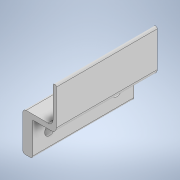
# Autodesk Inventor part: CableChain_Holder
Saved by Autodesk Inventor 2021 (Build 250183000, 183)
## iProperties
Created: 2021-12-04
Part Number: CableChain_Holder
Material: Generic
Document SubType Name: Modeling
Designer: Jorian Brusind
Density: 1 g/cm^3
Appearance: Default
Author: Jorian Brusind
Autodesk Inventor part; units mm, degrees
ref_plane "YZ Plane" through (0, 0, 0) normal (1, 0, 0) x (0, 1, 0)
ref_plane "XZ Plane" through (0, 0, 0) normal (0, 1, 0) x (-1, 0, 0)
ref_plane "XY Plane" through (0, 0, 0) normal (0, 0, 1) x (1, 0, 0)
sketch "Sketch1" plane through (0, 0, 0) normal (0, 1, 0) x (-1, 0, 0)
  line L0 (0, 0) -> (20, 0)
  line L1 (20, 0) -> (20, -60)
  line L2 (20, -60) -> (0, -60)
  line L3 (0, -60) -> (0, 0)
  dimension "d0" = 20
  dimension "d1" = 60
  constraints: 8 end point, 2 parallel, 1 horizontal, 1 perpendicular
  measures "d0" distance of L1.end L2.end
  measures "d1" distance of L0.end L1.end
extrude "Extrusion1" add sketch "Sketch1" along normal blind 3
sketch "Sketch2" plane through (0, 3, 0) normal (0, 1, 0) x (1, 0, 0)
  line L0 (-20, 0) -> (0, 0) projected
  line L1 (0, 0) -> (-2, 0)
  line L2 (-2, 0) -> (-2, 60)
  line L3 (-2, 60) -> (0, 60)
  line L4 (0, 60) -> (0, 0)
  dimension "d4" = 2
  dimension "d5" = 60
  constraints: 8 end point, 2 parallel, 1 horizontal, 1 perpendicular
  measures "d4" distance of L2.end L3.end
  measures "d5" distance of L1.end L2.end
extrude "Extrusion2" add sketch "Sketch2" along normal blind 22
sketch "Sketch3" plane through (0, 0, 0) normal (0, -1, 0) x (1, 0, 0)
  line L0 (-20, 0) -> (0, 0) projected
  line L1 (0, -60) -> (-20, -60) projected
  line L2 (-20, 0) -> (-14, 0)
  line L3 (-14, 0) -> (-14, -60)
  line L4 (-14, -60) -> (-20, -60)
  line L5 (-20, -60) -> (-20, 0)
  point P0 (-14, 0)
  dimension "d8" = 6
  constraints: 8 end point, 2 parallel, 1 horizontal, 1 perpendicular, 1 point on line
  measures "d8" distance of L3.end L4.end
extrude "Extrusion3" add sketch "Sketch3" along normal blind 20
sketch "Sketch4" plane through (-14, 0, 0) normal (1, 0, 0) x (0, 0, -1)
  line L0 (0, -20) -> (0, 0) projected
  line L1 (0, -10) -> (10, -10)
  line L2 (60, 0) -> (60, -20) projected
  circle A0 centre (10, -10) radius 3
  line L3 (60, -20) -> (0, -20) projected
  line L4 (0, -20) -> (60, -20)
  circle A1 centre (50, -10) radius 3
  point P0 (0, 3)
  point P1 (-60, -3)
  dimension "d11" = 10
  dimension "d12" = 6
  dimension "d15" = 40
  constraints: 4 end point, 2 centre point, 2 horizontal, 1 coincident, 1 collinear, 1 midpoint, 3 other
  measures "d11" distance of L1.start L1.end
  measures "d12" diameter of A0
  measures "d15" distance of A0.centre A1.centre
extrude "Extrusion4" cut sketch "Sketch4" against normal through all
fillet "Fillet3" radius 3 2 edges at (-2, 3, -30) (0, 0, -30)
fillet "Fillet4" radius 1 2 edges at (0, 25, -30) (-2, 25, -30)
fillet "Fillet6" radius 1.5 2 edges at (-20, -20, -30) (-14, -20, -30)
fillet "Fillet10" radius 2 1 edges at (-20, 3, -30)
body "Solid1"
